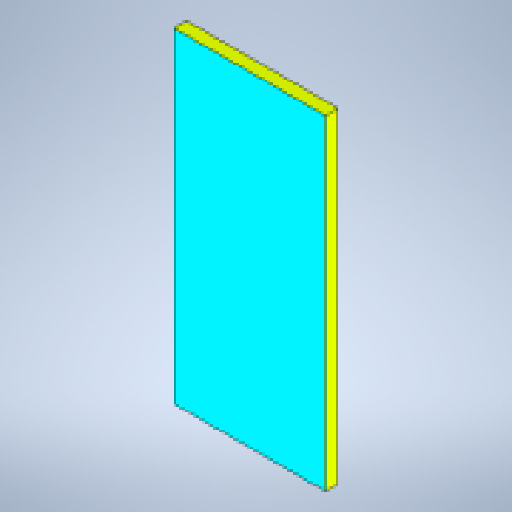
# Autodesk Inventor part: GnG- -Sandwich wall low
Saved by Autodesk Inventor 2025.3 (Build 293356000, 356)
## iProperties
Created: 2023-05-28
Part Number: GnG- -Sandwich wall low
Material: Generic
Document SubType Name: Modeling
Designer: admin
Density: 1 g/cm^3
Appearance: Default
Author: user
Autodesk Inventor part; units mm, degrees
ref_plane "YZ Plane" through (0, 0, 0) normal (1, 0, 0) x (0, 1, 0)
ref_plane "XZ Plane" through (0, 0, 0) normal (0, 1, 0) x (-1, 0, 0)
ref_plane "XY Plane" through (0, 0, 0) normal (0, 0, 1) x (1, 0, 0)
sketch "Sketch1" plane through (0, 0, 0) normal (0, 0, 1) x (1, 0, 0)
  line L0 (0, 0) -> (1200, 0)
  line L1 (1200, 0) -> (1200, 2570)
  line L2 (1200, 2570) -> (0, 2570)
  line L3 (0, 2570) -> (0, 0)
  dimension "d0" = 1200
  dimension "d1" = 2570
  constraints: 8 end point, 2 parallel, 1 horizontal, 1 perpendicular
  measures "d0" distance of L2.end L1.end
  measures "d1" distance of L1.end L0.end
extrude "Extrusion1" add sketch "Sketch1" along normal blind 100
chamfer "Chamfer1" distance 2 angle 45 1 edges at (1200, 1285, 100)
body "Solid1"
